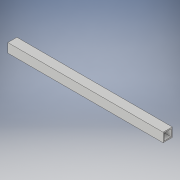
# Autodesk Inventor part: 17in 1x1 Beam
Saved by Autodesk Inventor 2018 (Build 220112000, 112)
## iProperties
Created: 2019-01-16
Part Number: 17in 1x1 Beam
Material: Generic
Document SubType Name: Modeling
Designer: Gabriel
Density: 1 g/cm^3
Appearance: Default
Author: Gabriel
Autodesk Inventor part; units mm, degrees
ref_plane "YZ Plane" through (0, 0, 0) normal (1, 0, 0) x (0, 1, 0)
ref_plane "XZ Plane" through (0, 0, 0) normal (0, 1, 0) x (-1, 0, 0)
ref_plane "XY Plane" through (0, 0, 0) normal (0, 0, 1) x (1, 0, 0)
sketch "Sketch1" plane through (0, 0, 0) normal (1, 0, 0) x (0, 1, 0)
  line L0 (4.2484, 4.9473) -> (-21.1516, 4.9473)
  line L1 (-21.1516, 4.9473) -> (-21.1516, -20.4527)
  line L2 (-21.1516, -20.4527) -> (4.2484, -20.4527)
  line L3 (4.2484, -20.4527) -> (4.2484, 4.9473)
  line L4 (1.0734, 1.7723) -> (-17.9766, 1.7723)
  line L5 (-17.9766, 1.7723) -> (-17.9766, -17.2777)
  line L6 (-17.9766, -17.2777) -> (1.0734, -17.2777)
  line L7 (1.0734, -17.2777) -> (1.0734, 1.7723)
  point P0 (0, 0)
  dimension "d0" = 25.4
  dimension "d1" = 25.4
  dimension "d2" = 3.175
  constraints: 16 end point, 4 parallel, 2 perpendicular, 1 horizontal, 3 other
  measures "d0" distance of L2.end L1.end
  measures "d1" distance of L1.end L0.end
  measures "d2" distance between parallel lines of L3 L7
extrude "Extrusion1" add sketch "Sketch1" along normal blind 431.8
body "Solid1"
